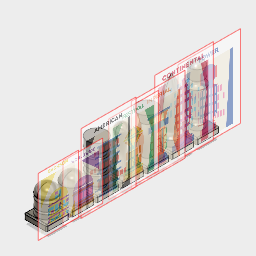
Acquire hotel markers v7 (Autodesk Fusion 360 design; units mm, degrees)
Autodesk Fusion 360 part; units mm, degrees
sketch "Sketch1" plane through (0, 0, 0) normal (0, 1, 0) x (1, 0, 0)
  line L0 (0, 0) -> (20, 0)
  line L1 (20, 0) -> (20, 20)
  line L2 (20, 20) -> (0, 20)
  line L3 (0, 20) -> (0, 0)
  line L4 (0, 0) -> (10, 0) construction
  line L5 (0, 0) -> (20, 20) construction
  line L6 (0, 20) -> (20, 0) construction
  line L7 (18, 2) -> (2, 2)
  line L8 (2, 2) -> (2, 18)
  line L9 (2, 18) -> (18, 18)
  line L10 (18, 18) -> (18, 2)
  line L11 (18, 2) -> (2, 18) construction
  line L12 (2, 2) -> (18, 18) construction
  point P0 (10, 10)
  dimension "d1" = 20
  dimension "d2" = 20
  dimension "d6" = 16
  dimension "d7" = 16
  measures "d1" distance of L0.start L2.end
  measures "d2" distance of L0.start L0.end
  measures "d6" distance of L8.end L9.end
  measures "d7" distance of L7.end L8.end
extrude "Extrude1" add sketch "Sketch1" along normal blind 3 makes body 1
sketch "Sketch2" plane through (0, 3, 0) normal (0, 1, 0) x (-1, 0, 0)
  line L0 (-2, -18) -> (-18, -18)
  line L1 (-18, -18) -> (-18, -2)
  line L2 (-18, -2) -> (-2, -2)
  line L3 (-2, -2) -> (-2, -18)
  line L4 (0, -20) -> (0, 0)
  line L5 (0, 0) -> (-20, 0)
  line L6 (-20, 0) -> (-20, -20)
  line L7 (-20, -20) -> (0, -20)
  line L8 (0, 0) -> (-20, 0)
  line L9 (-20, 0) -> (-20, -20)
  line L10 (-20, -20) -> (0, -20)
  line L11 (0, -20) -> (0, 0)
extrude "Extrude2" add sketch "Sketch2" along normal blind 2 contours L0 L1 L2 L3 | L4 L5 L6 L7 L8 L9 L10 L11 bodies 1
fillet "Fillet1" radius 1 8 edges at (0, 2.5, 0) (20, 2.5, 0) (20, 2.5, -20) (20, 5, -10) (10, 5, 0) (10, 5, -20) (0, 5, -10) (0, 2.5, -20) on bodies 1
pattern_linear "R-Pattern1" count 7 spacing 22 along (0, 0, 1) both ways of bodies 1 makes body 2 at (13, 5, -73) makes body 3 at (13, 5, -51) makes body 4 at (13, 5, -29) makes body 5 at (13, 5, 15) makes body 6 at (13, 5, 37) makes body 7 at (13, 5, 59)
sketch "Sketch3" plane through (0, 0, 0) normal (0, 0, 1) x (1, 0, 0)
sketch "Sketch4" plane through (0, 0, 0) normal (1, 0, 0) x (0, 0, -1)
ref_plane "WorkPlane1" through (10, 0, 0) normal (1, 0, 0) x (0, 1, 0)
sketch "Sketch5" plane through (10, 0, 0) normal (1, 0, 0) x (0, 0, -1)
  line L0 (-65, 5) -> (-47, 5)
  line L1 (-21, 5) -> (-3, 5)
  line L2 (63, 5) -> (45, 5)
  line L3 (-43, 5) -> (-25, 5)
  line L4 (1, 5) -> (19, 5)
  line L5 (23, 5) -> (41, 5)
  line L6 (85, 5) -> (67, 5)
  line L7 (-56, 5) -> (-65, 5)
  line L8 (-56, 5) -> (-56, 28.0109)
  line L9 (-64.1292, 5) -> (-64.1292, 8.982)
  spline S0 degree 5 poles (-56, 28.0109) (-56.2733, 28.0109) (-56.8092, 27.9968) (-57.5804, 27.9332) (-58.5469, 27.7651) (-59.6653, 27.4214) (-60.7053, 26.9457) (-61.6694, 26.333) (-62.5439, 25.57) (-63.295, 24.6343) (-63.877, 23.4971) (-64.1682, 22.4011) (-64.27, 21.462) (-64.2834, 20.7822) (-64.2765, 20.4288) knots 0 0 0 0 0 0 0.1 0.2 0.3 0.4 0.5 0.6 0.7 0.8 0.9 1 1 1 1 1 1
  line L10 (-64.3133, 22.3059) -> (-64.2397, 18.5517)
  line L11 (-54.3855, 28.0109) -> (-57.6145, 28.0109)
  line L12 (-64.1292, 10.8959) -> (-64.1292, 16.969)
  line L13 (-64.1292, 16.969) -> (-62.7674, 18.3676)
  line L14 (-62.7674, 18.3676) -> (-64.1292, 19.6936)
  line L15 (-64.1292, 19.6936) -> (-64.2765, 20.4288)
  line L16 (-64.1292, 8.982) -> (-63.0768, 10.0629)
  line L17 (-63.0768, 10.0629) -> (-64.1292, 10.8959)
  line L18 (-34, 5) -> (-34, 25.9537)
  line L19 (-42.7197, 5) -> (-42.7197, 18.6643)
  spline S1 degree 5 poles (-42.7197, 18.6643) (-42.6571, 18.947) (-42.5221, 19.5004) (-42.2904, 20.2948) (-41.9219, 21.2811) (-41.3555, 22.3844) (-40.6738, 23.3463) (-39.8673, 24.1554) (-38.9306, 24.8051) (-37.8689, 25.3016) (-36.6914, 25.6563) (-35.6644, 25.836) (-34.8493, 25.9158) (-34.2864, 25.9451) (-34, 25.9537) knots 0 0 0 0 0 0 0.1 0.2 0.3 0.4 0.5 0.6 0.7 0.8 0.9 1 1 1 1 1 1
  line L20 (-12, 5) -> (-12, 41.526)
  line L21 (-12, 41.526) -> (-20.4819, 41.526)
  line L22 (-20.4819, 41.526) -> (-20.4819, 34.0335)
  line L23 (-20.4819, 34.0335) -> (-18.3866, 31.7865)
  line L24 (-18.3866, 31.7865) -> (-18.3866, 28.9919)
  line L25 (-18.3866, 28.9919) -> (-20.4324, 28.9919)
  line L26 (-20.4324, 28.9919) -> (-20.4324, 21.4426)
  line L27 (-20.4819, 16.4033) -> (-20.4819, 8.9144)
  line L28 (-18.3866, 28.9919) -> (-18.3866, -3.1113) construction
  line L29 (-20.4819, 16.4033) -> (-18.3866, 16.4033)
  line L30 (-20.4324, 21.4426) -> (-18.3866, 19.2487)
  line L31 (-20.4819, 8.9144) -> (-18.3866, 6.6675)
  line L32 (-18.3866, 5) -> (-18.3866, 6.6675)
  line L33 (-18.3866, 16.4033) -> (-18.3866, 19.2487)
  line L34 (10, 5) -> (10, 40.7124)
  line L35 (10, 5) -> (2.5695, 5)
  line L36 (2.5695, 5) -> (2.5695, 8.8993)
  spline S2 degree 5 poles (2.5695, 8.8993) (2.6713, 9.1042) (2.8739, 9.5186) (3.1747, 10.1539) (3.5694, 11.0284) (4.0513, 12.1675) (4.5195, 13.3522) (4.9694, 14.5819) (5.3936, 15.8549) (5.7806, 17.1685) (6.1164, 18.5184) (6.3864, 19.8981) (6.5771, 21.2991) (6.6783, 22.7096) (6.6846, 24.1146) (6.5976, 25.4952) (6.4255, 26.8316) (6.1816, 28.106) (5.8845, 29.3065) (5.5566, 30.4292) (5.2244, 31.4828) (4.9166, 32.4876) (4.663, 33.4672) (4.4927, 34.4421) (4.4323, 35.4231) (4.5043, 36.4037) (4.7278, 37.3637) (5.1183, 38.2728) (5.6887, 39.0944) (6.4496, 39.7894) (7.4094, 40.3202) (8.3411, 40.5876) (9.1339, 40.6894) (9.7043, 40.7122) (10, 40.7124) knots 0 0 0 0 0 0 0.033333 0.066667 0.1 0.133333 0.166667 0.2 0.233333 0.266667 0.3 0.333333 0.366667 0.4 0.433333 0.466667 0.5 0.533333 0.566667 0.6 0.633333 0.666667 0.7 0.733333 0.766667 0.8 0.833333 0.866667 0.9 0.933333 0.966667 1 1 1 1 1 1
  line L37 (5.5584, 40.7101) -> (14.4416, 40.7146)
  line L38 (32, 5) -> (32, 40.8403)
  line L39 (32, 40.8403) -> (23.5394, 40.8403)
  line L40 (23.5394, 40.8403) -> (27.3604, 31.1884)
  spline S3 degree 5 poles (28.0594, 5) (27.7969, 5.5591) (27.3027, 6.6714) (26.6542, 8.3224) (25.9715, 10.4924) (25.4047, 13.1728) (25.1047, 15.8423) (25.0496, 18.515) (25.2139, 21.1907) (25.5617, 23.8434) (26.0535, 26.4308) (26.5346, 28.4113) (26.9338, 29.8285) (27.2156, 30.7405) (27.3604, 31.1884) knots 0 0 0 0 0 0 0.1 0.2 0.3 0.4 0.5 0.6 0.7 0.8 0.9 1 1 1 1 1 1
  line L41 (26.562, 28.7198) -> (28.1589, 33.657)
  line L42 (29.3952, 2.155) -> (26.7235, 7.845)
  line L43 (54, 5) -> (54, 56.6031)
  line L44 (54, 5) -> (46.3516, 5)
  line L45 (46.3516, 10.3119) -> (46.3516, 5)
  spline S4 degree 5 poles (46.3516, 10.3119) (46.6379, 10.4736) (47.1752, 10.8124) (47.8756, 11.3672) (48.5975, 12.1999) (49.1509, 13.3956) (49.3723, 14.7431) (49.3018, 16.2337) (49.0057, 17.8524) (48.5629, 19.58) (48.0542, 21.3948) (47.5513, 23.2745) (47.1047, 25.1981) (46.7458, 27.1471) (46.4913, 29.1069) (46.3473, 31.0686) (46.3127, 33.0299) (46.3835, 34.9977) (46.555, 36.9853) (46.8241, 39.0084) (47.1917, 41.081) (47.6643, 43.2121) (48.257, 45.4003) (48.9939, 47.6332) (49.9032, 49.8918) (51.014, 52.1542) (52.0846, 53.9506) (52.9983, 55.2833) (53.6577, 56.1644) (54, 56.6031) knots 0 0 0 0 0 0 0.04 0.08 0.12 0.16 0.2 0.24 0.28 0.32 0.36 0.4 0.44 0.48 0.52 0.56 0.6 0.64 0.68 0.72 0.76 0.8 0.84 0.88 0.92 0.96 1 1 1 1 1 1
  line L46 (50.6113, 52.2597) -> (57.3887, 60.9465)
  line L47 (76, 5) -> (76, 55.7875)
  line L48 (70.3737, 5) -> (70.3737, 8.9539)
  line L49 (68.4866, 15.5589) -> (68.4866, 37.2574)
  line L50 (69.7776, 43.1433) -> (69.7776, 52.0482)
  spline S5 degree 5 poles (69.7776, 52.0482) (69.8679, 52.1741) (70.0496, 52.421) (70.3259, 52.7769) (70.7029, 53.2234) (71.1976, 53.7382) (71.727, 54.2121) (72.3024, 54.6442) (72.9319, 55.0287) (73.617, 55.3538) (74.3563, 55.604) (74.9891, 55.7309) (75.4859, 55.7785) (75.827, 55.7882) (76, 55.7875) knots 0 0 0 0 0 0 0.1 0.2 0.3 0.4 0.5 0.6 0.7 0.8 0.9 1 1 1 1 1 1
  line L51 (69.2562, 51.3212) -> (70.2989, 52.7751)
  line L52 (75.0779, 55.7912) -> (76.9221, 55.7838)
  spline S6 degree 5 poles (69.7776, 43.1433) (69.9757, 43.0329) (70.3517, 42.8115) (70.8554, 42.4775) (71.4042, 42.028) (71.8722, 41.459) (72.1049, 40.8823) (72.0861, 40.2974) (71.813, 39.7041) (71.3016, 39.1029) (70.5724, 38.4946) (69.8303, 38.0027) (69.1904, 37.6311) (68.7273, 37.3822) (68.4866, 37.2574) knots 0 0 0 0 0 0 0.1 0.2 0.3 0.4 0.5 0.6 0.7 0.8 0.9 1 1 1 1 1 1
  spline S7 degree 5 poles (68.4866, 15.5589) (68.7366, 15.4447) (69.2185, 15.2147) (69.887, 14.8652) (70.668, 14.3898) (71.4471, 13.7791) (72.0103, 13.1501) (72.3377, 12.5013) (72.4146, 11.8314) (72.2452, 11.1407) (71.8459, 10.4307) (71.3563, 9.8483) (70.8994, 9.404) (70.5555, 9.1045) (70.3737, 8.9539) knots 0 0 0 0 0 0 0.1 0.2 0.3 0.4 0.5 0.6 0.7 0.8 0.9 1 1 1 1 1 1
  point P0 (-61.516, 26.3915)
  point P1 (-39.823, 24.1256)
  point P2 (5.0678, 14.897)
  point P3 (6.6566, 22.7614)
  point P4 (5.7033, 29.9109)
  point P5 (4.5118, 34.5184)
  point P6 (5.3061, 38.4904)
  point P7 (25.1148, 18.9235)
  point P8 (49.2619, 14.3556)
  point P9 (47.9752, 21.7079)
  point P10 (46.3516, 31.6947)
  point P11 (47.5165, 42.482)
  point P12 (72.2576, 54.5924)
  point P13 (72.0557, 40.4778)
  point P14 (72.3182, 12.3294)
  dimension "d35" = 137
  measures "d35" angle of L22 L23
revolve "Revolve3" add sketch "Sketch5" angle 360 about axis through (10, 5, 56) along (0, 1, 0) contours L0 L7 L8 L9 S0 L12 L13 L14 L15 L16 L17 bodies 7
revolve "Revolve4" add sketch "Sketch5" angle 360 about axis through (10, 5, 34) along (0, 1, 0) contours L3 L18 L19 S1 bodies 6
revolve "Revolve5" add sketch "Sketch5" angle 360 about axis through (10, 5, 12) along (0, 1, 0) contours L1 L20 L21 L22 L23 L24 L25 L26 L27 L29 L30 L31 L32 L33 bodies 5
revolve "Revolve6" add sketch "Sketch5" angle 360 about axis through (10, 5, -10) along (0, 1, 0) contours L4 L34 L35 L36 S2 bodies 1
revolve "Revolve7" add sketch "Sketch5" angle 360 about axis through (10, 5, -32) along (0, 1, 0) contours L5 L38 L39 L40 S3 bodies 4
revolve "Revolve8" add sketch "Sketch5" angle 360 about axis through (10, 5, -54) along (0, 1, 0) contours L2 L43 L44 L45 S4 bodies 3
revolve "Revolve9" add sketch "Sketch5" angle 360 about axis through (10, 5, -76) along (0, 1, 0) contours L6 L47 L48 L49 L50 S5 S6 S7 bodies 2
box "BoxPrimitive1" add length 164.3264 width 40.2245 height 10 placed x (0, 0, -1) y (-1, 0, 0) z (0, 1, 0) at (30.8086, 0, 71.008) separate body makes body 8
hidden bodies 8
named bodies: "Festival", "Tower", "Continental", "Imperial", "American", "Worldwide", "Sackson", "10mm modifier"
